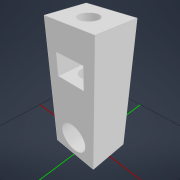
# Autodesk Inventor part: mgn_screw_nut
Saved by Autodesk Inventor 2022 (Build 260153000, 153)
## iProperties
Created: 2021-06-28
Part Number: mgn_screw_nut
Material: Generic
Document SubType Name: Modeling
Designer: user
Density: 1 g/cm^3
Appearance: Default
Author: user
Autodesk Inventor part; units mm, degrees
ref_plane "YZ Plane" through (0, 0, 0) normal (1, 0, 0) x (0, 1, 0)
ref_plane "XZ Plane" through (0, 0, 0) normal (0, 1, 0) x (-1, 0, 0)
sketch "Sketch1" plane through (0, 0, 0) normal (0, 0, 1) x (1, 0, 0)
  line L0 (-6, -5) -> (6, -5)
  line L1 (6, -5) -> (6, 5)
  line L2 (6, 5) -> (-6, 5)
  line L3 (-6, 5) -> (-6, -5)
  line L4 (-6, -5) -> (6, 5) construction
  line L5 (6, -5) -> (-6, 5) construction
  circle A0 centre (0, -0.25) radius 2.125
  point P0 (0, 0)
  point P1 (0, 0)
  point P2 (0, 0)
  dimension "d0" = 12
  dimension "d1" = 10
  dimension "d2" = 4.25
  dimension "d18" = 0.25
  constraints: 12 end point, 4 midpoint, 2 parallel, 1 centre point, 1 horizontal, 1 perpendicular, 1 vertical alignment, 1 other
  measures "d0" distance of L2.end L1.end
  measures "d1" distance of L1.end L0.end
  measures "d2" diameter of A0
  measures "d18" distance of point (0, 0) A0.centre
extrude "Extrusion1" add sketch "Sketch1" along normal blind 30
sketch "Sketch2" plane through (-6, -5, 0) normal (0, -1, 0) x (1, 0, 0)
  circle A0 centre (6, 5) radius 2.1
  line L0 (0, 0) -> (12, 0) projected
  point P0 (6, 0)
  point P1 (6, 0)
  dimension "d5" = 4.2
  dimension "d6" = 5
  constraints: 1 centre point, 1 midpoint, 1 vertical alignment
  measures "d5" diameter of A0
  measures "d6" distance from line of L0 A0.centre
sketch "Sketch3" plane through (0, 0, 0) normal (0, 0, -1) x (-1, 0, 0)
  line L0 (-6, -5) -> (-6, 5) projected
  line L1 (6, -5) -> (-6, -5) projected
  line L2 (6, 5) -> (6, -5) projected
  line L3 (-6, 5) -> (6, 5) projected
  circle A0 centre (0, -0.25) radius 2.125 projected
  point P0 (0, 0)
extrude "Extrusion2" add sketch "Sketch3" against normal blind 10 contours A0
extrude "Extrusion3" cut sketch "Sketch2" against normal through all
ref_plane "Work Plane1" through (0, 0, 24) normal (0, 0, 1) x (1, 0, 0)
sketch "Sketch4" plane through (0, 0, 24) normal (0, 0, 1) x (1, 0, 0)
  line L0 (3.475, -2.0063) -> (0, -4.0126) construction
  line L1 (0, -4.0126) -> (-3.475, -2.0063) construction
  line L2 (-3.475, -2.0063) -> (-3.475, 2.0063)
  line L3 (-3.475, 2.0063) -> (0, 4.0126)
  line L4 (0, 4.0126) -> (3.475, 2.0063)
  line L5 (3.475, 2.0063) -> (3.475, -2.0063)
  line L6 (3.475, -2.0063) -> (3.475, -9.9564)
  line L7 (-3.475, -2.0063) -> (-3.475, -9.9564)
  line L8 (-3.475, -9.9564) -> (3.475, -9.9564)
  point P0 (0, 0)
  point P1 (0, 0)
  dimension "d12" = 6.95
  constraints: 18 end point, 3 vertical, 1 coincident, 1 perpendicular, 13 other
  measures "d12" distance between parallel lines of L5 L2
extrude "Extrusion4" cut sketch "Sketch4" against normal blind 5
sketch "Sketch5" plane through (-6, -5, 0) normal (0, -1, 0) x (1, 0, 0)
  circle A0 centre (6, 5) radius 2.1 projected
  circle A1 centre (6, 5) radius 3.625
  point P0 (6, 0)
  dimension "d15" = 7.25
  constraints: 1 centre point, 1 coincident
  measures "d15" diameter of A1
extrude "Extrusion5" cut sketch "Sketch5" against normal blind 4
body "Solid1"
